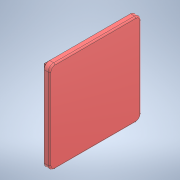
# Autodesk Inventor part: cube-inlay-red
Saved by Autodesk Inventor 2020 (Build 240168000, 168)
## iProperties
Created: 2019-11-16
Part Number: cube-inlay-red
Material: Generic
Document SubType Name: Modeling
Designer: Paul Koch
Density: 1 g/cm^3
Appearance: Default
Author: Paul Koch
Autodesk Inventor part; units mm, degrees
ref_plane "YZ Plane" through (0, 0, 0) normal (1, 0, 0) x (0, 1, 0)
ref_plane "XZ Plane" through (0, 0, 0) normal (0, 1, 0) x (-1, 0, 0)
ref_plane "XY Plane" through (0, 0, 0) normal (0, 0, 1) x (1, 0, 0)
sketch "Sketch1" plane through (0, 0, 0) normal (1, 0, 0) x (0, 1, 0)
  line L0 (-7.5, 8.5) -> (7.5, 8.5)
  line L1 (8.5, 7.5) -> (8.5, -7.5)
  line L2 (7.5, -8.5) -> (-7.5, -8.5)
  line L3 (-8.5, -7.5) -> (-8.5, 7.5)
  line L4 (-8.5, 8.5) -> (8.5, -8.5) construction
  line L5 (8.5, 8.5) -> (-8.5, -8.5) construction
  line L6 (-7.5, 7.5) -> (7.5, 7.5)
  line L7 (7.5, 7.5) -> (7.5, -7.5)
  line L8 (7.5, -7.5) -> (-7.5, -7.5)
  line L9 (-7.5, -7.5) -> (-7.5, 7.5)
  line L10 (-7.5, 7.5) -> (7.5, -7.5) construction
  line L11 (7.5, 7.5) -> (-7.5, -7.5) construction
  line L12 (-5.5, 5.5) -> (5.5, 5.5)
  line L13 (5.5, 5.5) -> (5.5, -5.5)
  line L14 (5.5, -5.5) -> (-5.5, -5.5)
  line L15 (-5.5, -5.5) -> (-5.5, 5.5)
  line L16 (-5.5, 5.5) -> (5.5, -5.5) construction
  line L17 (5.5, 5.5) -> (-5.5, -5.5) construction
  arc A0 (8.5, 7.5) -> (7.5, 8.5) centre (7.5, 7.5) ccw
  arc A1 (-7.5, 8.5) -> (-8.5, 7.5) centre (-7.5, 7.5) ccw
  arc A2 (-8.5, -7.5) -> (-7.5, -8.5) centre (-7.5, -7.5) ccw
  arc A3 (7.5, -8.5) -> (8.5, -7.5) centre (7.5, -7.5) ccw
  point P0 (0, 0)
  dimension "d0" = 17
  dimension "d1" = 17
  dimension "d2" = 15
  dimension "d3" = 15
  dimension "d4" = 11
  dimension "d5" = 11
  dimension "d12" = 1
  constraints: 36 end point, 8 point on circle, 8 point on line, 8 tangent, 6 midpoint, 6 parallel, 4 centre point, 3 equal radius, 3 horizontal, 3 perpendicular
  measures "d0" distance of L4.end L5.end
  measures "d1" distance of L5.start L4.end
  measures "d2" distance of L7.end L8.end
  measures "d3" distance of L6.end L7.end
  measures "d4" distance of L13.end L14.end
  measures "d5" distance of L12.end L13.end
  measures "d12" radius of A0
extrude "Extrusion3" add sketch "Sketch1" along normal blind 1 contours L0 A0 L1 A3 L2 A2 L3 A1 | L6 L7 L8 L9 | L12 L13 L14 L15
extrude "Extrusion4" add sketch "Sketch1" against normal blind 1 contours L6 L7 L8 L9
fillet "Fillet3" radius 0.25 8 edges at (1, 8.2071, 8.2071) (1, 0, 8.5) (1, -8.2071, 8.2071) (1, -8.5, 0) (1, -8.2071, -8.2071) (1, 0, -8.5) (1, 8.2071, -8.2071) (1, 8.5, 0)
body "Solid2"
